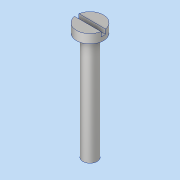
# Autodesk Inventor part: M1.6x0.35 Bolt
Saved by Autodesk Inventor 2017 SP1 (Build 210196100, 196)
## iProperties
Created: 2019-01-01
Part Number: M1.6x0.35 Bolt
Material: Aluminum 6061
Document SubType Name: Modeling
Designer: Dylan Rice
Density: 2.7 g/cm^3
Appearance: Aluminum - Flat
Author: Dylan Rice
Autodesk Inventor part; units mm, degrees
ref_plane "YZ Plane" through (0, 0, 0) normal (1, 0, 0) x (0, 1, 0)
ref_plane "XZ Plane" through (0, 0, 0) normal (0, 1, 0) x (-1, 0, 0)
ref_plane "XY Plane" through (0, 0, 0) normal (0, 0, 1) x (1, 0, 0)
sketch "Sketch1" plane through (0, 0, 0) normal (0, 1, 0) x (-1, 0, 0)
  circle A0 centre (0, 0) radius 0.8
  dimension "d0" = 1.6
  constraints: 1 centre point, 1 coincident
  measures "d0" diameter of A0
extrude "Extrusion1" add sketch "Sketch1" along normal blind 13
sketch "Sketch2" plane through (0, 13, 0) normal (0, 1, 0) x (1, 0, 0)
  circle A0 centre (0, 0) radius 0.8 projected
  circle A1 centre (0, 0) radius 1.5
  dimension "d3" = 3
  constraints: 1 centre point, 1 coincident
  measures "d3" diameter of A1
extrude "Extrusion2" add sketch "Sketch2" against normal blind 1
sketch "Sketch3" plane through (0, 13, 0) normal (0, 1, 0) x (1, 0, 0)
  line L0 (2, -0.25) -> (-2, -0.25)
  line L1 (-2, -0.25) -> (-2, 0.25)
  line L2 (-2, 0.25) -> (2, 0.25)
  line L3 (2, 0.25) -> (2, -0.25)
  line L4 (2, -0.25) -> (-2, 0.25) construction
  line L5 (-2, -0.25) -> (2, 0.25) construction
  point P0 (0, 0)
  dimension "d6" = 0.5
  dimension "d7" = 4
  constraints: 12 end point, 2 midpoint, 2 parallel, 1 horizontal, 1 perpendicular
  measures "d6" distance between parallel lines of L2 L0
  measures "d7" distance between parallel lines of L1 L3
extrude "Extrusion3" cut sketch "Sketch3" against normal blind 0.5
body "Solid1"
